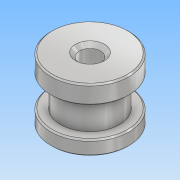
# Autodesk Inventor part: втулка фитинг
Saved by Autodesk Inventor 2017 (Build 210142000, 142)
## iProperties
Part Number: втулка фитинг
Material: Типовые
Document SubType Name: Modeling
Designer: STALKER
Density: 1 g/cm^3
Appearance: Алюминий — полированный
Author: STALKER
Autodesk Inventor part; units mm, degrees
ref_plane "YZ Plane" through (0, 0, 0) normal (1, 0, 0) x (0, 1, 0)
ref_plane "XZ Plane" through (0, 0, 0) normal (0, 1, 0) x (-1, 0, 0)
ref_plane "XY Plane" through (0, 0, 0) normal (0, 0, 1) x (1, 0, 0)
sketch "Эскиз1" plane through (0, 0, 0) normal (0, 0, 1) x (1, 0, 0)
  line L0 (0, 0) -> (0, 15) construction
  line L1 (0, 0) -> (-22, 0) construction
  circle A0 centre (0, 0) radius 2.15
  circle A1 centre (0, 0) radius 8
  circle A2 centre (0, 0) radius 6
  circle A3 centre (0, 0) radius 5
  dimension "d0" = 4.3
  dimension "d1" = 16
  dimension "d2" = 12
  dimension "d3" = 10
  constraints: 4 centre point, 4 coincident, 4 end point, 1 vertical
  measures "d0" diameter of A0
  measures "d1" diameter of A1
  measures "d2" diameter of A2
  measures "d3" diameter of A3
extrude "Выдавливание1" add sketch "Эскиз1" along normal blind 3.8 contours A1 | A2 | A3
extrude "Выдавливание2" add sketch "Эскиз1" against normal blind 9 contours A1 | A2
extrude "Выдавливание3" cut sketch "Эскиз1" against normal blind 6 contours A1
extrude "Выдавливание4" add sketch "Эскиз1" against normal blind 2.2 contours A3
chamfer "Фаска1" distance 2.85 distance2 1 1 edges at (-2.15, 0, -2.2) measured on face at (4.0016, -0.3989, -2.2)
sketch "Эскиз2" plane through (0, 0, -9) normal (0, 0, -1) x (-1, 0, 0)
  circle A0 centre (0, 0) radius 5
  circle A1 centre (0, 0) radius 3.25
  dimension "d15" = 10
  dimension "d16" = 6.5
  constraints: 2 centre point, 2 coincident
  measures "d15" diameter of A0
  measures "d16" diameter of A1
extrude "Выдавливание5" add sketch "Эскиз2" along normal blind 0.5 and the other way blind 2
chamfer "Фаска2" distance 0.8 angle 45 1 edges at (3.25, 0, -9.5)
fillet "Сопряжение1" radius 0.1 1 edges at (5, 0, -9.5)
chamfer "Фаска3" distance 0.8 angle 45 1 edges at (-2.15, 0, 3.8)
chamfer "Фаска4" distance 0.3 angle 45 4 edges at (-8, 0, 3.8) (-8, 0, 0) (-8, 0, -6) (-8, 0, -9)
